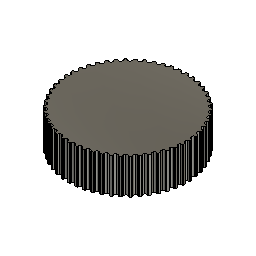
gear_54z (Autodesk Fusion 360 design; units mm, degrees)
Autodesk Fusion 360 part; units mm, degrees
sketch "Sketch1" plane through (0, 0, 0) normal (0, 0, 1) x (1, 0, 0) in component "gt2 pulley"
  circle A0 centre (0, 0) radius 17.1887 construction
  circle A1 centre (0, 0) radius 16.1847 construction
  line L0 (0, 0) -> (0, 17.1887) construction
  line L1 (0, 0) -> (0.9994, 17.1597) construction
  line L2 (0, 0) -> (1.4068, 17.1311) construction
  circle A2 centre (0, 0) radius 16.9347 construction
  arc A3 (0.3894, 16.7954) -> (0.4586, 16.5037) centre (1.386, 16.8779) ccw
  circle A4 centre (0, 0) radius 16.7847 construction
  arc A5 (0.242, 16.933) -> (0, 16.9347) centre (0, 0) ccw
  arc A6 (0.3894, 16.7954) -> (0.242, 16.933) centre (0.2399, 16.783) ccw
  arc A7 (0.4586, 16.5037) -> (0.9411, 16.1574) centre (0.9733, 16.7114) ccw
  arc A8 (0, 16.9347) -> (-0.242, 16.933) centre (0, 0) ccw
  arc A9 (-0.242, 16.933) -> (-0.3894, 16.7954) centre (-0.2399, 16.783) ccw
  arc A10 (-0.4586, 16.5037) -> (-0.3894, 16.7954) centre (-1.386, 16.8779) ccw
  arc A11 (-0.9413, 16.1573) -> (-0.4586, 16.5037) centre (-0.9733, 16.7114) ccw
  arc A12 (0.9411, 16.1574) -> (-0.9411, 16.1574) centre (0, 0) ccw
  point P0 (1.386, 16.8779)
  point P1 (0, 16.9347)
  dimension "d18" = 34.3775
  dimension "d19" = 3.333
  dimension "d22" = 1.004
  dimension "d24" = 0.75
  dimension "d26" = 1
  dimension "d27" = 0.15
  dimension "d28" = 0.15
  dimension "d47" = 0.555
  dimension "d52" = 3.812
  constraint coincident A0.centre A1.centre
  constraint coincident A0 L0.end
  constraint vertical L0
  constraint coincident A0 L1.end
  constraint coincident A0 L2.end
  constraint concentric A1 A2
  constraint coincident A1 A7.end
  constraint coincident L1 A7.end
  constraint coincident A2 P0
  constraint coincident L2 P0
  constraint coincident P0 A3.centre
  constraint coincident A2 P1
  constraint coincident L0 P1
  constraint concentric A2 A4
  constraint coincident P1 A5.end
  constraint coincident A4 A6.centre
  constraint coincident A3.start A6.start
  constraint tangent A3 A6
  constraint tangent A3 A7
  constraint symmetric L0 A7.end A12.end
  constraint symmetric L0 A3.start A9.end
  constraint symmetric L0 A3.end A10.start
  constraint symmetric L0 A3 A10
  constraint symmetric L0 A5.start A8.end
  constraint symmetric L0 P1 A5.end
  constraint symmetric L0 A5 A8
  constraint symmetric L0 A6 A9
  constraint symmetric L0 A7 A11
  constraint coincident A1 A11.start
  constraint tangent A1 A7
  constraint coincident L1 A7.centre
  measures "d18" diameter of A0
  measures "d19" angle of L0 L1
  measures "d22" distance of A0 A1
  measures "d24" distance of A1 A2
  measures "d26" radius of A3
  measures "d27" distance of A2 A4
  measures "d28" radius of A6
  measures "d47" radius of A7
extrude "Extrude1" add sketch "Sketch1" along normal blind 10 makes body 1
pattern_circular "C-Pattern1" count 54 over 360 about axis through (0, 0, 1.75) along (0, 0, 1) of bodies 1 makes body 2 at (-1.9829, 16.0628, 6.6667) makes body 3 at (-3.8343, 15.724, 6.6667) makes body 4 at (-5.6338, 15.1725, 6.6667) makes body 5 at (-7.3571, 14.4159, 6.6667) makes body 6 at (-8.2729, 13.9106, 6.6667) makes body 7 at (-10.4834, 12.3306, 6.6667) makes body 8 at (-11.844, 11.0302, 6.6667) makes body 9 at (-13.4061, 9.0676, 6.6667) makes body 10 at (-14.0685, 8.0015, 6.6667) makes body 11 at (-14.5559, 7.0761, 6.6667) makes body 12 at (-15.6468, 4.1382, 6.6667) makes body 13 at (-15.7954, 3.5285, 3.3333) makes body 14 at (-16.0982, 1.6709, 6.6667) makes body 15 at (-16.1185, -1.4629, 6.6667) makes body 16 at (-16.0497, -2.0866, 6.6667) makes body 17 at (-15.6989, -3.9358, 6.6667) makes body 18 at (-14.5558, -7.0763, 6.6667) makes body 19 at (-13.9637, -8.1829, 6.6667) makes body 20 at (-13.406, -9.0677, 6.6667) makes body 21 at (-12.2627, -10.5628, 6.6667) makes body 22 at (-10.9535, -11.915, 6.6667) makes body 23 at (-8.2727, -13.9107, 6.6667) makes body 24 at (-7.9105, -14.1198, 6.6667) makes body 25 at (-6.2178, -14.9427, 6.6667) makes body 26 at (-4.441, -15.5635, 6.6667) makes body 27 at (-2.6041, -15.9739, 6.6667) makes body 28 at (0.1047, -16.1844, 6.6667) makes body 29 at (2.6043, -15.9738, 6.6667) makes body 30 at (3.8343, -15.724, 6.6667) makes body 31 at (4.8419, -15.4435, 6.6667) makes body 32 at (7.9107, -14.1197, 6.6667) makes body 33 at (8.2729, -13.9106, 6.6667) makes body 34 at (9.8319, -12.8561, 6.6667) makes body 35 at (11.844, -11.0302, 6.6667) makes body 36 at (13.4061, -9.0676, 6.6667) makes body 37 at (14.0685, -8.0015, 6.6667) makes body 38 at (14.9023, -6.3141, 6.6667) makes body 39 at (15.5345, -4.5414, 6.6667) makes body 40 at (15.7954, -3.5285, 6.6667) makes body 41 at (16.0982, -1.6709, 3.3333) makes body 42 at (16.1509, 1.0456, 6.6667) makes body 43 at (16.0497, 2.0866, 6.6667) makes body 44 at (15.6989, 3.9358, 6.6667) makes body 45 at (14.5558, 7.0763, 6.6667) makes body 46 at (13.6359, 8.7183, 6.6667) makes body 47 at (13.406, 9.0677, 6.6667) makes body 48 at (12.2627, 10.5628, 6.6667) makes body 49 at (10.9535, 11.915, 6.6667) makes body 50 at (8.806, 13.5794, 6.6667) makes body 51 at (7.1699, 14.5099, 6.6667) makes body 52 at (4.8417, 15.4436, 6.6667) makes body 53 at (3.0161, 15.9012, 6.6667) makes body 54 at (2.6041, 15.9739, 6.6667)
sketch "Sketch2" plane through (0, 0, 10) normal (0, 0, 1) x (-1, 0, 0)
  arc A0 (-9.5546, -13.8184) -> (-9.507, -14.0143) centre (-9.4229, -13.8902) ccw
  arc A1 (-9.507, -14.0143) -> (-9.1026, -14.2803) centre (0, 0) ccw
  arc A2 (-9.1026, -14.2803) -> (-8.9039, -14.2463) centre (-9.022, -14.1538) ccw
  arc A3 (-8.6858, -14.0407) -> (-8.9039, -14.2463) centre (-8.1166, -14.8629) ccw
  arc A4 (-8.0924, -14.0164) -> (-8.6858, -14.0407) centre (-8.3699, -14.497) ccw
  arc A5 (-9.6649, -12.9822) -> (-8.0924, -14.0164) centre (0, 0) ccw
  arc A6 (-9.4521, -13.5366) -> (-9.6649, -12.9822) centre (-9.9963, -13.4273) ccw
  arc A7 (-9.5546, -13.8184) -> (-9.4521, -13.5366) centre (-10.4326, -13.3397) ccw
  circle A8 centre (0, 0) radius 16.1847
  constraint concentric A1 A8
extrude "Extrude2" add sketch "Sketch2" against normal blind 10 contours A5 A8 bodies 1 2 3 4 5 6 7 8 9 10 11 12 13 14 15 16 17 18 19 20 21 22 23 24 25 26 27 28 29 30 31 32 33 34 35 36 37 38 39 40 41 42 43 44 45 46 47 48 49 50 51 52 53 54
extrude "Extrude4" [suppressed] in component "gt2 pulley"
pattern_circular "C-Pattern7" [suppressed] in component "gt2 pulley"
extrude "Extrude3" [suppressed] in component "gt2 pulley"
pattern_circular "C-Pattern6" [suppressed] in component "gt2 pulley"
extrude "Extrude2'" [suppressed] in component "gt2 pulley"
pattern_circular "C-Pattern5" [suppressed] in component "gt2 pulley"
extrude "Extrude1'" [suppressed] in component "gt2 pulley"
pattern_circular "C-Pattern4" [suppressed] in component "gt2 pulley"
pattern_circular "C-Pattern3" [suppressed] in component "gt2 pulley"
pattern_circular "C-Pattern2" [suppressed] in component "gt2 pulley"
pattern_circular "C-Pattern1'" [suppressed] in component "gt2 pulley"
copy_body "Body->Comp1" [suppressed] in component "Component"
copy_body "Body->Comp2" [suppressed] in component "Component'"
copy_body "Body->Comp3" [suppressed] in component "Component''"
copy_body "Body->Comp4" [suppressed] in component "Component'''"
copy_body "Body->Comp5" [suppressed] in component "Component''''"
copy_body "Body->Comp6" [suppressed] in component "Component'''''"
copy_body "Body->Comp7" [suppressed] in component "Component''''''"
copy_body "Body->Comp8" [suppressed] in component "Component'''''''"
copy_body "Body->Comp9" [suppressed] in component "Component''''''''"
copy_body "Body->Comp10" [suppressed] in component "Component'''''''''"
copy_body "Body->Comp11" [suppressed] in component "Component''''''''''"
copy_body "Body->Comp12" [suppressed] in component "Component'''''''''''"
copy_body "Body->Comp13" [suppressed] in component "Component''''''''''''"
copy_body "Body->Comp14" [suppressed] in component "Component'''''''''''''"
copy_body "Body->Comp15" [suppressed] in component "Component''''''''''''''"
copy_body "Body->Comp16" [suppressed] in component "Component'''''''''''''''"
copy_body "Body->Comp17" [suppressed] in component "Component''''''''''''''''"
copy_body "Body->Comp18" [suppressed] in component "Component'''''''''''''''''"
copy_body "Body->Comp19" [suppressed] in component "Component''''''''''''''''''"
copy_body "Body->Comp20" [suppressed] in component "Component'''''''''''''''''''"
component "gt2 pulley" placed x (1, 0, 0) y (0, 1, 0) z (0, 0, 1) at (0, 0, 0)
equation "NumTeeth = 54" comment "min 20"
equation "ToothPitch = 2 mm"
equation "PullyDia = NumTeeth * ToothPitch / PI"
equation "ToothAng = ( ( 360 / NumTeeth ) * 1 deg )"
equation "TransOffsetAngle = ToothAng * 0.2"
equation "Sholulder_Radius = 0.15 mm"
equation "Root_Radius = 0.555 mm"
equation "TransRadius = 1 mm"
equation "ToolHeight = 0.75 mm"
equation "PLD = 0.254 mm"
equation "d18 = PullyDia"
equation "d19 = ToothAng / 2"
equation "d22 = PLD + ToolHeight"
equation "d24 = ToolHeight"
equation "d26 = TransRadius"
equation "d27 = Sholulder_Radius"
equation "d31 = NumTeeth"
equation "d33 = NumTeeth"
equation "d35 = NumTeeth"
equation "d37 = NumTeeth"
equation "d41 = NumTeeth"
equation "d45 = NumTeeth"
equation "d47 = Root_Radius"
equation "d50 = NumTeeth"
